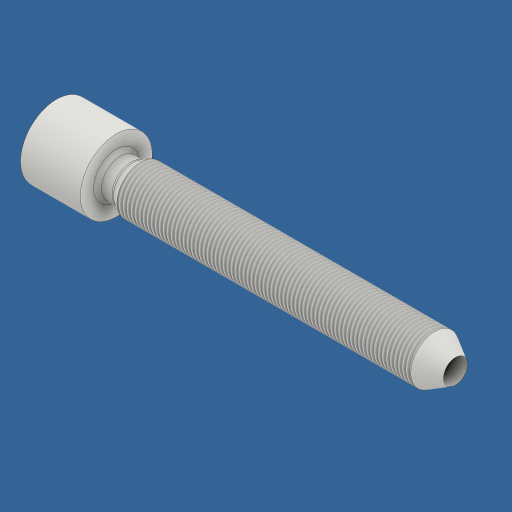
# Autodesk Inventor part: 2.3_Druckschraube
Saved by Autodesk Inventor 2024.3 (Build 283343000, 343)
## iProperties
Created: 2025-09-05
Part Number: 2.3_Druckschraube
Material: 1.0038 S235JR
Document SubType Name: Modeling
Designer: klose.julius
Density: 7.86 g/cm^3
Appearance: Stahl
Author: klose.julius
Autodesk Inventor part; units mm, degrees
ref_plane "YZ Plane" through (0, 0, 0) normal (1, 0, 0) x (0, 1, 0)
ref_plane "XZ Plane" through (0, 0, 0) normal (0, 1, 0) x (-1, 0, 0)
ref_plane "XY Plane" through (0, 0, 0) normal (0, 0, 1) x (1, 0, 0)
sketch "Skizze1" plane through (0, 0, 0) normal (0, 0, 1) x (1, 0, 0)
  line L0 (-35, 0) -> (105, 0) projected
  line L1 (0, -1.8) -> (0, 10.8) projected
  line L2 (0, 0) -> (65, 0)
  line L3 (85, 0) -> (85, 3)
  line L4 (79.8038, 6) -> (6.1517, 6)
  line L5 (0, 6) -> (0, 0)
  line L6 (0, 0) -> (-15, 0)
  line L7 (-15, 0) -> (-15, 9)
  line L8 (-15, 9) -> (0, 9)
  line L9 (0, 9) -> (0, 0)
  line L10 (85, 0) -> (65, 0)
  line L11 (85, 3) -> (85, 0)
  line L12 (85, 3) -> (79.8038, 6)
  line L13 (0, 0) -> (3.9, 0)
  line L14 (3.9, 0) -> (3.9, 4.7)
  line L15 (3.9, 4.7) -> (0, 4.7)
  line L16 (0, 4.7) -> (0, 0)
  line L17 (3.9, 4.7) -> (6.1517, 6)
  point P0 (85, 1.5)
  point P1 (0, 4.7)
  dimension "d2" = 9
  dimension "d3" = 100
  dimension "d7" = 30
  dimension "d8" = 12
  dimension "d10" = 6
  dimension "d11" = 85
  dimension "d12" = 9.4
  dimension "d13" = 3.9
  dimension "d17" = 30
  constraints: 32 end point, 7 parallel, 4 horizontal, 3 perpendicular, 1 coincident, 1 midpoint
  measures "d2" distance of L6.end L7.end
  measures "d3" distance between parallel lines of L3 L7
  measures "d7" angle of L4 L12
  measures "d8" diameter of L4 L0
  measures "d10" diameter of L3.end L0
  measures "d11" distance from line of point (85, 1.5) L1
  measures "d12" diameter of L15 L0
  measures "d13" distance between parallel lines of L14 L5
  measures "d17" angle of L4 L17
revolve "Umdrehung1" add sketch "Skizze1" angle 360 about axis through (-10, 0, 0) along (1, 0, 0)
sketch "Skizze2" plane through (85, 0, 0) normal (1, 0, 0) x (0, 0, -1)
  point P0 (0, 0)
  point P1 (0, 0)
  constraints: 1 coincident
hole "Bohrung1" at (85, 0, 0) direction (-1, 0, 0) diameter 6 depth 20 tip angle 118
fillet "Rundung1" radius 1 1 edges at (0, -4.7, 0)
fillet "Rundung2" radius 1 1 edges at (3.9, -4.7, 0)
thread "Gewinde1" size "M12x1" class "6g" standard "ANSI Metric M Profile" full length
sketch "Skizze3" plane through (-15, 0, 0) normal (-1, 0, 0) x (0, 0, 1)
  point P0 (0, 0)
